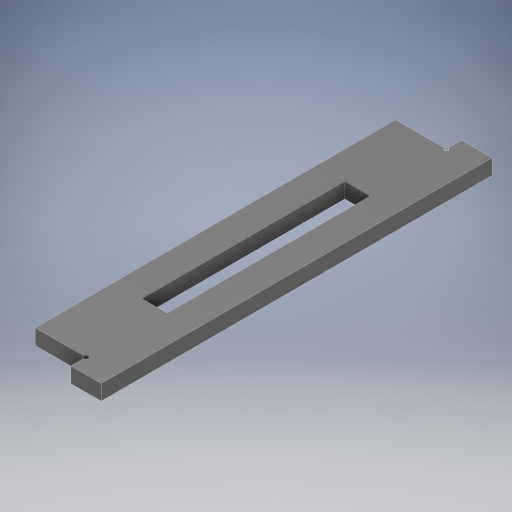
# Autodesk Inventor part: battery bottomplate
Saved by Autodesk Inventor 2024 (Build 280153000, 153)
## iProperties
Created: 2024-09-04
Part Number: battery bottomplate
Material: PMMA 플라스틱
Document SubType Name: Modeling
Designer: msi
Density: 1.188 g/cm^3
Appearance: 매끄러움 - 검은색
Author: msi
Autodesk Inventor part; units mm, degrees
ref_plane "우측면도" through (0, 0, 0) normal (1, 0, 0) x (0, 1, 0)
ref_plane "평면도" through (0, 0, 0) normal (0, 1, 0) x (-1, 0, 0)
ref_plane "정면도" through (0, 0, 0) normal (0, 0, 1) x (1, 0, 0)
sketch "스케치1" plane through (0, 0, 0) normal (0, 1, 0) x (-1, 0, 0)
  line L0 (-16, 71) -> (16, 71)
  line L1 (16, 71) -> (16, -71)
  line L2 (16, -71) -> (-16, -71)
  line L3 (-16, -71) -> (-16, 71)
  line L4 (-16, 71) -> (16, -71) construction
  line L5 (16, 71) -> (-16, -71) construction
  line L6 (-16, -71) -> (-4, -71)
  line L7 (-4, -71) -> (-4, -77)
  line L8 (-4, -77) -> (-16, -77)
  line L9 (-16, -77) -> (-16, -71)
  line L10 (-16, 71) -> (-4, 71)
  line L11 (-4, 71) -> (-4, 77)
  line L12 (-4, 77) -> (-16, 77)
  line L13 (-16, 77) -> (-16, 71)
  point P0 (0, 0)
  dimension "d0" = 32
  dimension "d1" = 142
  dimension "d2" = 12
  dimension "d3" = 6
  dimension "d4" = 12
  dimension "d5" = 6
  constraints: 28 end point, 6 parallel, 3 horizontal, 3 perpendicular, 2 midpoint
  measures "d0" distance of L1.end L2.end
  measures "d1" distance of L0.end L1.end
  measures "d2" distance of L7.end L8.end
  measures "d3" distance of L6.end L7.end
  measures "d4" distance of L12.end L11.end
  measures "d5" distance of L11.end L10.end
extrude "돌출1" add sketch "스케치1" along normal blind 6
sketch "스케치2" plane through (0, 6, 0) normal (0, 1, 0) x (1, 0, 0)
  line L0 (-5, -40) -> (5, -40)
  line L1 (5, -40) -> (5, 40)
  line L2 (5, 40) -> (-5, 40)
  line L3 (-5, 40) -> (-5, -40)
  line L4 (-5, -40) -> (5, 40) construction
  line L5 (5, -40) -> (-5, 40) construction
  point P0 (0, 0)
  dimension "d8" = 10
  dimension "d9" = 80
  constraints: 12 end point, 2 midpoint, 2 parallel, 1 horizontal, 1 perpendicular
  measures "d8" distance of L2.end L1.end
  measures "d9" distance of L1.end L0.end
extrude "돌출2" cut sketch "스케치2" against normal blind 6
sketch "스케치3" plane through (0, 6, 0) normal (0, 1, 0) x (1, 0, 0)
  line L0 (-5, 40) -> (5, 40) projected
  line L1 (5, 40) -> (5, -40) projected
  line L2 (5, -40) -> (-5, -40) projected
  line L3 (-5, -40) -> (-5, 40) projected
  line L4 (-16, -71) -> (4, -71) projected
  line L5 (4, -71) -> (4, -77) projected
  line L6 (4, -77) -> (16, -77) projected
  line L7 (16, -77) -> (16, 77) projected
  line L8 (16, 77) -> (4, 77) projected
  line L9 (4, 77) -> (4, 71) projected
  line L10 (4, 71) -> (-16, 71) projected
  line L11 (-16, 71) -> (-16, -71) projected
  circle A0 centre (4, -71) radius 1
  circle A1 centre (4, 71) radius 1
  point P0 (0, 0)
  dimension "d12" = 2
  dimension "d13" = 2
  constraints: 2 centre point, 2 coincident
  measures "d12" diameter of A0
  measures "d13" diameter of A1
extrude "돌출3" cut sketch "스케치3" against normal through all contours A0 L5 L4 | L4 L5 A0 | A1 L9 L10 | L10 L9 A1
